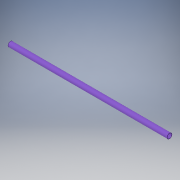
# Autodesk Inventor part: Front Idler roller
Saved by Autodesk Inventor 2017 (Build 210142000, 142)
## iProperties
Created: 2017-01-14
Part Number: Front Idler roller
Material: Generic
Document SubType Name: Modeling
Designer: Ben
Density: 1 g/cm^3
Appearance: Violet
Author: Ben
Autodesk Inventor part; units mm, degrees
ref_plane "YZ Plane" through (0, 0, 0) normal (1, 0, 0) x (0, 1, 0)
ref_plane "XZ Plane" through (0, 0, 0) normal (0, 1, 0) x (-1, 0, 0)
ref_plane "XY Plane" through (0, 0, 0) normal (0, 0, 1) x (1, 0, 0)
sketch "Sketch1" plane through (0, 0, 0) normal (1, 0, 0) x (0, 1, 0)
  circle A0 centre (0, 0) radius 9.525
  circle A1 centre (0, 0) radius 8.7313
  dimension "d0" = 19.05
  dimension "d4" = 0.7937
  constraints: 2 centre point, 2 coincident
  measures "d0" diameter of A0
  measures "d4" radial gap between concentric circles of A0 A1
extrude "Extrusion1" add sketch "Sketch1" along normal mid plane 603.25
body "Solid1"
